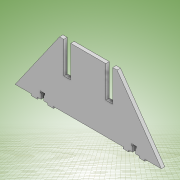
# Autodesk Inventor part: UnionColumnas
Saved by Autodesk Inventor 2022 (Build 260153000, 153)
## iProperties
Created: 2022-02-24
Part Number: UnionColumnas
Material: Genérico
Document SubType Name: Modeling
Designer: Marco
Density: 1 g/cm^3
Appearance: Valor por defecto
Author: Marco
Autodesk Inventor part; units mm, degrees
ref_plane "YZ Plane" through (0, 0, 0) normal (1, 0, 0) x (0, 1, 0)
ref_plane "XZ Plane" through (0, 0, 0) normal (0, 1, 0) x (-1, 0, 0)
ref_plane "XY Plane" through (0, 0, 0) normal (0, 0, 1) x (1, 0, 0)
sketch "Boceto1" plane through (0, 0, 0) normal (0, 0, 1) x (1, 0, 0)
  line L0 (254.0457, 0) -> (177.0228, 110)
  line L1 (77.0228, 110) -> (0, 0)
  line L2 (84.5228, 110) -> (84.5228, 55)
  line L3 (84.5228, 55) -> (96.5228, 55)
  line L4 (96.5228, 55) -> (96.5228, 110)
  line L5 (157.5228, 110) -> (157.5228, 55)
  line L6 (157.5228, 55) -> (169.5228, 55)
  line L7 (169.5228, 55) -> (169.5228, 110)
  line L8 (84.5228, 110) -> (77.0228, 110)
  line L9 (177.0228, 110) -> (169.5228, 110)
  line L10 (157.5228, 110) -> (96.5228, 110)
  line L11 (0, 0) -> (40.0401, 0)
  line L12 (40.0401, 0) -> (254.0457, 0)
  dimension "d1" = 100
  dimension "d2" = 110
  dimension "d3" = 61
  dimension "d5" = 12
  dimension "d6" = 7.5
  dimension "d12" = 55
  dimension "d23" = 55
  dimension "d24" = 55
  constraints: 26 end point, 8 horizontal alignment, 2 equal length, 2 horizontal, 2 parallel, 1 point on line, 1 vertical alignment
  measures "d1" distance of L0.end L1.start
  measures "d2" vertical distance of L1.end L1.start
  measures "d3" distance of L5.end L3.end
  measures "d5" distance of L2.end L3.end
  measures "d6" distance of L1.start L2.start
  measures "d12" distance of L2.start L2.end
  measures "d23" angle of L11 L1
  measures "d24" angle of L12 L0
extrude "Extrusión1" add sketch "Boceto1" along normal blind 6
sketch "Boceto3" plane through (0, 0, 6) normal (0, 0, 1) x (1, 0, 0)
  line L0 (0, 0) -> (254.0457, 0) projected
  line L1 (50, 9) -> (50, 0)
  line L2 (45, 0) -> (45, 9)
  line L3 (43.5, 12) -> (51.5, 12)
  line L4 (51.5, 12) -> (51.5, 9)
  line L5 (43.5, 9) -> (43.5, 12)
  line L6 (51.5, 9) -> (50, 9)
  line L7 (45, 9) -> (43.5, 9)
  line L8 (157.5228, 110) -> (96.5228, 110) projected
  line L9 (127.0228, 110) -> (127.0228, 0)
  line L10 (204.0457, 9) -> (204.0457, 0)
  line L11 (209.0457, 0) -> (209.0457, 9)
  line L12 (210.5457, 12) -> (202.5457, 12)
  line L13 (202.5457, 12) -> (202.5457, 9)
  line L14 (210.5457, 9) -> (210.5457, 12)
  line L15 (202.5457, 9) -> (204.0457, 9)
  line L16 (209.0457, 9) -> (210.5457, 9)
  line L17 (45, 0) -> (50, 0) construction
  line L18 (204.0457, 0) -> (209.0457, 0) construction
  point P0 (204.0457, 0)
  point P1 (47.5, 12)
  point P2 (47.5, 0)
  point P3 (206.5457, 0)
  dimension "d25" = 5
  dimension "d26" = 8
  dimension "d27" = 12
  dimension "d29" = 45
  dimension "d30" = 3
  constraints: 34 end point, 8 symmetric about line, 5 midpoint, 4 parallel, 3 vertical alignment, 2 horizontal, 2 point on line, 1 collinear, 1 horizontal alignment, 1 perpendicular
  measures "d25" distance of L1.end L2.start
  measures "d26" distance of L3.start L3.end
  measures "d27" vertical distance of L3.start L2.start
  measures "d29" distance of L2.start L0.start
  measures "d30" distance of L3.end L4.end
extrude "Extrusión3" cut sketch "Boceto3" against normal up to next
sketch "Boceto4" plane through (0, 0, 0) normal (0, -1, 0) x (1, 0, 0)
  line L0 (77.0228, 6) -> (0, 6) projected
  line L1 (77.0228, 0) -> (0, 0) projected
  line L2 (38.5114, 6) -> (28.5114, 6)
  line L3 (28.5114, 6) -> (28.5114, 0)
  line L4 (28.5114, 0) -> (38.5114, 0)
  line L5 (38.5114, 0) -> (38.5114, 6)
  line L6 (50, 0) -> (204.0457, 0) projected
  line L7 (56.5114, 6) -> (66.5114, 6)
  line L8 (66.5114, 6) -> (66.5114, 0)
  line L9 (66.5114, 0) -> (56.5114, 0)
  line L10 (56.5114, 0) -> (56.5114, 6)
  line L11 (157.5228, 0) -> (96.5228, 0) projected
  line L12 (127.0228, 0) -> (127.0228, 6) construction
  line L13 (215.5342, 6) -> (225.5342, 6)
  line L14 (225.5342, 6) -> (225.5342, 0)
  line L15 (225.5342, 0) -> (215.5342, 0)
  line L16 (215.5342, 0) -> (215.5342, 6)
  line L17 (197.5342, 6) -> (187.5342, 6)
  line L18 (187.5342, 6) -> (187.5342, 0)
  line L19 (187.5342, 0) -> (197.5342, 0)
  line L20 (197.5342, 0) -> (197.5342, 6)
  dimension "d33" = 10
  dimension "d34" = 18
  dimension "d35" = 10
  constraints: 34 end point, 8 symmetric about line, 4 parallel, 3 point on line, 2 horizontal, 2 midpoint, 2 perpendicular, 1 vertical
  measures "d33" distance of L4.end L3.end
  measures "d34" distance of L9.end L4.end
  measures "d35" distance of L9.end L8.end
extrude "Extrusión4" add sketch "Boceto4" along normal blind 3 contours L8 L1 L10 L0 | L5 L1 L3 L0 | L18 L17 L20 L6 | L13 L14 L15 L16
